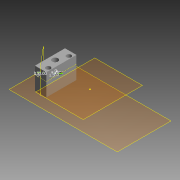
# Autodesk Inventor part: OPENSTOPBRKT
Saved by Autodesk Inventor 2015 (Build 190159000, 159)
## iProperties
Created: 2015-09-18
Part Number: OPENSTOPBRKT
Material: Generic
Description: insert part description/title
Document SubType Name: Modeling
Designer: francis
Density: 1 g/cm^3
Appearance: Default
Part Category: insert part category here and press enter to fill value
Author: francis
Autodesk Inventor part; units mm, degrees
ref_plane "YZ Plane" through (0, 0, 0) normal (1, 0, 0) x (0, 1, 0)
ref_plane "XZ Plane" through (0, 0, 0) normal (0, 1, 0) x (-1, 0, 0)
ref_plane "XY Plane" through (0, 0, 0) normal (0, 0, 1) x (1, 0, 0)
ref_plane "Work Plane1" through (0, 0, 0) normal (0, 0, 1) x (1, 0, 0)
sketch "Sketch1" plane through (0, 0, 0) normal (0, 0, 1) x (1, 0, 0)
  circle A0 centre (-27.5, 9) radius 2 projected
  circle A1 centre (-27.5, -9) radius 2 projected
  circle A2 centre (-30.5, 0) radius 2.5 projected
  line L0 (-25, 13.1624) -> (-25, -12.5061)
  line L1 (-35, -13.1624) -> (-35, 13.1624) projected
  line L2 (-25, -12.5061) -> (-25, -13.1624)
  line L3 (-25, -13.1624) -> (-35, -13.1624)
  line L4 (-35, 13.1624) -> (-25, 13.1624)
  arc A3 (-2.9901, -1.4163) -> (-18.371, -4.3253) centre (-12.371, 6.067) ccw construction
  point P0 (0, 0)
  dimension "d31" = 2.5
  constraints: 8 end point, 2 point on circle, 2 vertical, 1 centre point, 1 horizontal, 1 perpendicular
  measures "d31" distance from line of L0 A0.centre
ref_plane "Work Plane2" through (-37, -13, 19) normal (0, 0, -1) x (0, 1, 0)
extrude "Extrusion1" add sketch "Sketch1" along normal up to surface (19 mm away)
ref_plane "Work Plane3" through (-0.8627, 0, 12) normal (0, 0, 1) x (1, 0, 0)
sketch "Sketch4" plane through (-0.8627, 0, 12) normal (0, 0, 1) x (1, 0, 0)
  circle A0 centre (-29.6373, 0) radius 2.5 construction
  circle A1 centre (-26.6373, -9) radius 2 construction
  circle A2 centre (-26.6373, 9) radius 2 construction
  line L0 (-34.1373, -13.1624) -> (-24.1373, -13.1624) construction
  line L1 (-24.1373, -13.1624) -> (-24.1373, 13.1624) construction
  line L2 (-24.1373, 13.1624) -> (-34.1373, 13.1624) construction
  line L3 (-34.1373, 13.1624) -> (-34.1373, -13.1624) construction
  line L4 (-24.1373, 13.1624) -> (-24.1373, -13.1624) construction
  line L5 (-24.1373, -2.5647) -> (-34.1373, -10.9557) construction
  line L6 (-34.1373, -13.1624) -> (-34.1373, 13.1624) construction
  line L7 (-24.1373, -0.6066) -> (-34.1373, -8.9976) construction
  line L8 (-24.1373, 1.3515) -> (-34.1373, -7.0395) construction
  line L9 (-23.1842, 0.1932) -> (-35.6373, -10.2562)
  point P0 (0.8627, 0)
  dimension "d7" = 130
  dimension "d8" = 1.5
  dimension "d9" = 1.5
  dimension "d10" = 0
  dimension "d13" = 1.5
  constraints: 8 end point, 7 point on line, 2 parallel
  measures "d7" angle of L3 L5
  measures "d8" distance between parallel lines of L8 L7
  measures "d9" distance between parallel lines of L5 L7
  measures "d10" distance edge to line of A0 L8
  measures "d13" distance from line of L3 L9.end
ref_plane "Work Plane6" through (-35, -7.0395, 12) normal (-0.7660444, -0.6427876, 0) x (0.6427876, -0.7660444, 0)
sketch "Sketch7" plane through (-35, -7.0395, 12) normal (-0.7660444, -0.6427876, 0) x (0.6427876, -0.7660444, 0)
  point P0 (17.105, -12)
  point P1 (1.5, 0)
  point P2 (1.5, 0)
  point P3 (1.5, 0)
hole "Hole1" at (-34.0358, -8.1885, 12) direction (0.7660444, 0.6427876, 0) diameter 2.459 end through all thread size "M3x0.5" class "6H" standard "ISO Metric profile"
hole "Hole2" at (-34.0358, -8.1885, 12) direction (-0.7660444, -0.6427876, 0) diameter 2.459 end through all thread size "M3x0.5" class "6H" standard "ISO Metric profile"
body "Solid1"
